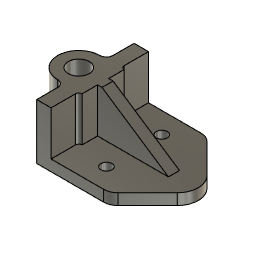
A3 (Autodesk Fusion 360 design; units mm, degrees)
Autodesk Fusion 360 part; units mm, degrees
note: some values were not read from the file. Set by a fixed rule: which sketch regions a step uses.
sketch "base" plane through (0, 0, 0) normal (0, 0, 1) x (1, 0, 0)
  line L0 (49.5, 44) -> (-49.5, 44)
  line L1 (-49.5, 44) -> (-49.5, -44)
  line L2 (-49.5, -44) -> (49.5, -44)
  line L3 (49.5, -44) -> (49.5, 44)
  line L4 (49.5, 44) -> (-49.5, -44) construction
  line L5 (-49.5, 44) -> (49.5, -44) construction
  dimension "d1" = 99
  dimension "d2" = 88
  constraint horizontal L0
  constraint perpendicular L0 L1
  constraint parallel L0 L2
  constraint parallel L1 L3
  constraint coincident L4 origin
  constraint coincident L5 origin
  measures "d1" distance of L1.end L2.end
  measures "d2" distance of L0.end L1.end
extrude "Extrude1" add sketch "base" along normal blind 10
sketch "top" plane through (0, 0, 10) normal (0, 0, 1) x (-1, 0, 0)
  line L0 (-49.5, 44) -> (-49.5, -44)
  line L1 (-49.5, -44) -> (49.5, -44)
  line L2 (49.5, -44) -> (49.5, 44)
  line L3 (49.5, 44) -> (-49.5, 44)
  line L4 (49.5, 44) -> (36.5, 44)
  line L5 (36.5, 44) -> (36.5, -44)
  line L6 (36.5, -44) -> (49.5, -44)
  line L7 (49.5, -44) -> (49.5, 44)
  dimension "d5" = 13
  dimension "d6" = 88
  constraint horizontal L4
  constraint vertical L5
  constraint horizontal L6
  constraint vertical L7
  constraint coincident L2.end L3.start
  measures "d5" distance of L2.end L4.end
  measures "d6" distance of L2.end L1.end
extrude "Extrude2" add sketch "top" along normal blind 40 contours L1 L2 L3 L4 L5 L6 L7
sketch "circles" plane through (0, 0, 10) normal (0, 0, 1) x (-1, 0, 0)
  line L0 (36.5, -44) -> (36.5, 44)
  line L1 (36.5, 44) -> (-49.5, 44)
  line L2 (-49.5, 44) -> (-49.5, -44)
  line L3 (-49.5, -44) -> (36.5, -44)
  line L4 (36.5, 44) -> (5.5, 44) construction
  line L5 (36.5, -44) -> (5.5, -44) construction
  line L6 (5.5, -44) -> (5.5, 44) construction
  line L7 (5.5, 44) -> (5.5, 25) construction
  line L8 (5.5, -44) -> (5.5, -25) construction
  circle A0 centre (5.5, -25) radius 5
  circle A1 centre (5.5, 25) radius 5
  dimension "d9" = 31
  dimension "d10" = 31
  dimension "d11" = 19
  dimension "d12" = 19
  dimension "d13" = 10
  dimension "d14" = 10
  constraint coincident L0.end L1.start
  constraint perpendicular L0 L4
  constraint coincident L0.start L3.end
  constraint perpendicular L0 L5
  constraint coincident L6 L7.end
  constraint perpendicular L3 L8
  constraint coincident L8.end A0.centre
  constraint coincident L7.end A1.centre
  measures "d9" distance of L0.end L4.end
  measures "d10" distance of L0.start L5.end
  measures "d11" distance of L4.end L7.end
  measures "d12" distance of L5.end L8.end
  measures "d13" diameter of A0
  measures "d14" diameter of A1
extrude "Extrude3" cut sketch "circles" against normal blind 25 contours A0 | A1
sketch "back big rectangle" plane through (-36.5, 0, 0) normal (1, 0, 0) x (0, 1, 0)
  line L0 (-44, 10) -> (44, 10)
  line L1 (44, 10) -> (44, 50)
  line L2 (44, 50) -> (-44, 50)
  line L3 (-44, 50) -> (-44, 10)
  line L4 (0, 50) -> (-19, 50)
  line L5 (-19, 50) -> (-19, 10)
  line L6 (-19, 10) -> (19, 10)
  line L7 (0, 50) -> (19, 50)
  line L8 (19, 50) -> (19, 10)
  dimension "d17" = 19
  constraint midpoint L2 L4.start
  constraint coincident L0 L5.end
  constraint perpendicular L0 L5
  constraint coincident L0 L6.end
  constraint coincident L2 L7.end
  constraint perpendicular L0 L8
  measures "d17" distance of L4.start L4.end
extrude "Extrude4" add sketch "back big rectangle" along normal blind 3 contours L0 L2 L4 L5 L6 L7 L8
fillet "Fillet1" radius 3 2 edges at (-36.5, 19, 30) (-36.5, -19, 30)
sketch "back small rectangle" plane through (-33.5, 0, 0) normal (1, 0, 0) x (0, 1, 0)
  line L0 (19, 50) -> (-19, 50)
  line L1 (-19, 50) -> (-19, 10)
  line L2 (-19, 10) -> (19, 10)
  line L3 (19, 10) -> (19, 50)
  line L4 (5, 50) -> (5, 10)
  line L5 (5, 10) -> (-5, 10)
  line L6 (-5, 10) -> (-5, 50)
  line L7 (-5, 50) -> (5, 50)
  constraint coincident L0 L4.start
  constraint coincident L2 L4.end
  constraint perpendicular L2 L4
  constraint coincident L2 L5.end
  constraint coincident L0 L6.end
  constraint perpendicular L0 L6
extrude "Extrude5" add sketch "back small rectangle" along normal blind 4 contours L0 L2 L4 L5 L6 L7
sketch "triangle" plane through (0, 0, 0) normal (0, 1, 0) x (1, 0, 0)
  line L0 (-29.5, -50) -> (-29.5, -10)
  line L1 (-29.5, -10) -> (30.5, -10)
  line L2 (30.5, -10) -> (-29.5, -50)
  dimension "d50" = 60
  constraint vertical L0
  constraint perpendicular L0 L1
  measures "d50" distance of L0.end L1.end
extrude "Extrude7" add sketch "triangle" along normal mid plane 10
extrude "Extrude8" cut 1 faces at (49.5, -14.6667, 3.3333) along direction (-1, 0, 0) blind 16
extrude "Extrude9" add 1 faces at (33.5, -14.6667, 3.3333) along direction (1, 0, 0) blind 19
sketch "bIg circle corner" plane through (0, 0, 10) normal (0, 0, 1) x (-1, 0, 0)
  circle A0 centre (5.5, -25) radius 5
  line L0 (-30.5, 5) -> (33.5, 5)
  line L1 (33.5, 5) -> (33.5, 19)
  arc A1 (33.5, 19) -> (36.5, 22) centre (33.5, 22) ccw
  line L2 (36.5, 22) -> (36.5, 44)
  line L3 (36.5, 44) -> (-52.5, 44)
  line L4 (-52.5, 44) -> (-52.5, -44)
  line L5 (-52.5, -44) -> (36.5, -44)
  line L6 (36.5, -44) -> (36.5, -22)
  arc A2 (36.5, -22) -> (33.5, -19) centre (33.5, -22) ccw
  line L7 (33.5, -19) -> (33.5, -5)
  line L8 (33.5, -5) -> (-30.5, -5)
  circle A3 centre (5.5, 25) radius 5
  circle A4 centre (-33.5, 0) radius 19 construction
  line L9 (-30.5, -5) -> (-30.5, 5)
  dimension "d35" = 38
  measures "d35" diameter of A4
chamfer "Chamfer1" distance 36.13 angle 45 2 edges at (52.5, -44, 5) (52.5, 44, 5)
fillet "Fillet2" radius 19 2 edges at (52.5, -7.87, 5) (52.5, 7.87, 5)
fillet "Fillet3" radius 13 2 edges at (16.37, -44, 5) (16.37, 44, 5)
sketch "outside back rectangle" plane through (-49.5, 0, 0) normal (-1, 0, 0) x (0, -1, 0)
  line L0 (-44, 0) -> (44, 0)
  line L1 (44, 0) -> (44, 50)
  line L2 (44, 50) -> (-44, 50)
  line L3 (-44, 50) -> (-44, 0)
  line L4 (-44, 0) -> (-19, 0) construction
  line L5 (44, 0) -> (19, 0) construction
  line L6 (-19, 0) -> (-19, 50)
  line L7 (19, 0) -> (19, 50)
  line L8 (-19, 50) -> (19, 50)
  line L9 (-19, 0) -> (19, 0)
  dimension "d40" = 25
  dimension "d41" = 25
  constraint coincident L0.start L3.end
  constraint perpendicular L3 L4
  constraint coincident L0.end L1.start
  constraint perpendicular L1 L5
  constraint coincident L2 L6.end
  constraint perpendicular L2 L6
  constraint coincident L2 L7.end
  constraint perpendicular L2 L7
  measures "d40" distance of L0.start L4.end
  measures "d41" distance of L0.end L5.end
extrude "Extrude10" add sketch "outside back rectangle" along normal blind 25 contours L0 L2 L6 L7 L8 L9
fillet "Fillet4" radius 6 2 edges at (-49.5, -19, 25) (-49.5, 19, 25)
fillet "Fillet5" radius 19 2 edges at (-74.5, -19, 25) (-74.5, 19, 25)
sketch "top back circle" plane through (0, 0, 50) normal (0, 0, 1) x (-1, 0, 0)
  arc A0 (55.5, -19) -> (55.5, 19) centre (55.5, 0) ccw
  arc A1 (49.5, 25) -> (55.5, 19) centre (55.5, 25) ccw
  line L0 (49.5, 25) -> (49.5, 44)
  line L1 (49.5, 44) -> (36.5, 44)
  line L2 (36.5, 44) -> (36.5, 22)
  arc A2 (33.5, 19) -> (36.5, 22) centre (33.5, 22) ccw
  line L3 (33.5, 19) -> (33.5, 5)
  line L4 (33.5, 5) -> (29.5, 5)
  line L5 (29.5, -5) -> (33.5, -5)
  line L6 (33.5, -5) -> (33.5, -19)
  arc A3 (36.5, -22) -> (33.5, -19) centre (33.5, -22) ccw
  line L7 (36.5, -22) -> (36.5, -44)
  line L8 (36.5, -44) -> (49.5, -44)
  line L9 (49.5, -44) -> (49.5, -25)
  arc A4 (55.5, -19) -> (49.5, -25) centre (55.5, -25) ccw
  line L10 (29.5, 0) -> (55.5, 0) construction
  circle A5 centre (55.5, 0) radius 9.5
  line L11 (29.5, 5) -> (29.5, -5)
  dimension "d46" = 26
  dimension "d47" = 19
  constraint perpendicular L6 L10
  constraint coincident A0.centre L10.end
  measures "d46" distance of L10.start A0.centre
  measures "d47" diameter of A5
extrude "Extrude11" cut sketch "top back circle" against normal blind 65 contours A5
equation "d1 = 13 mm + 67 mm + 19 mm"
equation "d46 = 4 mm + 3 mm + 13 mm + 6 mm"
named bodies: "A3"
